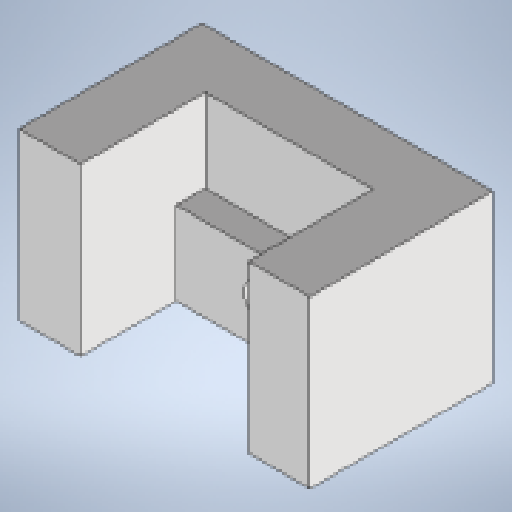
# Autodesk Inventor part: MotorMount
Saved by Autodesk Inventor 2026 (Build 300175050, 175E)
## iProperties
Created: 2025-12-25
Part Number: MotorMount
Material: Generic
Document SubType Name: Modeling
Designer: Nicholas M
Density: 1 g/cm^3
Appearance: Default
Author: Nicholas M
Autodesk Inventor part; units mm, degrees
ref_plane "YZ Plane" through (0, 0, 0) normal (1, 0, 0) x (0, 1, 0)
ref_plane "XZ Plane" through (0, 0, 0) normal (0, 1, 0) x (-1, 0, 0)
ref_plane "XY Plane" through (0, 0, 0) normal (0, 0, 1) x (1, 0, 0)
sketch "Sketch1" plane through (0, 16.25, -25.5) normal (1, 0, 0) x (0, 1, 0)
  line L0 (-35, 11.3959) -> (0, 11.3959)
  line L1 (0, 11.3959) -> (0, 41.3959)
  line L2 (0, 41.3959) -> (-35, 41.3959)
  line L3 (-35, 41.3959) -> (-35, 11.3959)
  line L4 (-17.5, 1.3959) -> (0, 1.3959)
  line L5 (-35, 41.3959) -> (0, 11.3959) construction
  line L6 (-35, 11.3959) -> (0, 41.3959) construction
  line L7 (-17.5, 53) -> (-17.5, 1.3959)
  circle A0 centre (-17.5, 16.3959) radius 2
  line L8 (-35, 26.3959) -> (0, 26.3959)
  line L9 (0, 26.3959) -> (0, 41.3959)
  line L10 (0, 41.3959) -> (-35, 41.3959)
  line L11 (-35, 41.3959) -> (-35, 26.3959)
  line L12 (-35, 11.3959) -> (-27.6, 11.3959)
  line L13 (-27.6, 11.3959) -> (-27.6, 41.3959)
  line L14 (-27.6, 41.3959) -> (-35, 41.3959)
  line L15 (-35, 41.3959) -> (-35, 11.3959)
  line L16 (0, 11.3959) -> (-7.4, 11.3959)
  line L17 (-7.4, 11.3959) -> (-7.4, 41.3959)
  line L18 (-7.4, 41.3959) -> (0, 41.3959)
  line L19 (0, 41.3959) -> (0, 11.3959)
  line L20 (0, 1.3959) -> (0, 49)
  line L21 (0, 31.3959) -> (0, 11.3959)
  line L22 (0, 11.3959) -> (0, 11.3959)
  line L23 (0, 11.3959) -> (0, 41.3959)
  line L24 (-35, 21.3959) -> (0, 21.3959)
  line L25 (-35, 18.8959) -> (-27.6, 18.8959)
  line L26 (-7.4, 18.8959) -> (0, 18.8959)
  line L27 (-35, 18.8959) -> (-27.6, 11.3959) construction
  line L28 (-35, 11.3959) -> (-27.6, 18.8959) construction
  circle A1 centre (-31.3, 15.1459) radius 1.625
  line L29 (-7.4, 11.3959) -> (0, 18.8959) construction
  line L30 (0, 11.3959) -> (-7.4, 18.8959) construction
  circle A2 centre (-3.7, 15.1459) radius 1.625
  line L31 (-35, 41.3959) -> (-27.6, 41.3959)
  line L32 (-27.6, 41.3959) -> (-27.6, 48.8959)
  line L33 (-27.6, 48.8959) -> (-35, 48.8959)
  line L34 (-35, 48.8959) -> (-35, 41.3959)
  line L35 (0, 41.3959) -> (-7.4, 41.3959)
  line L36 (-7.4, 41.3959) -> (-7.4, 48.8959)
  line L37 (-7.4, 48.8959) -> (0, 48.8959)
  line L38 (0, 48.8959) -> (0, 41.3959)
  line L39 (-35, 41.3959) -> (-27.6, 48.8959) construction
  line L40 (-35, 48.8959) -> (-27.6, 41.3959) construction
  line L41 (-7.4, 41.3959) -> (0, 48.8959) construction
  line L42 (-7.4, 48.8959) -> (0, 41.3959) construction
  circle A3 centre (-3.7, 45.1459) radius 1.625
  circle A4 centre (-31.3, 45.1459) radius 1.625
  circle A5 centre (-31.3, 30.1459) radius 2
  circle A6 centre (-3.7, 30.1459) radius 2
  line L43 (-27.6, 18.8959) -> (-35, 41.3959) construction
  line L44 (-35, 18.8959) -> (-27.6, 41.3959) construction
  point P0 (-17.5, 41.3959)
  point P1 (-17.5, 26.3959)
  point P2 (-1.25, 11.3959)
  point P3 (-27.6, 26.3959)
  point P4 (-7.4, 26.3959)
  point P5 (-7.4, 41.3959)
  point P6 (-7.4, 11.3959)
  point P7 (-27.6, 11.3959)
  point P8 (-17.5, 41.3959)
  point P9 (-17.5, 11.3959)
  point P10 (-1.25, 11.3959)
  point P11 (-7.4, 21.3959)
  point P12 (-27.6, 21.3959)
  point P13 (0, 21.3959)
  point P14 (0, 41.3959)
  point P15 (-3.7, 15.1459)
  dimension "d5" = 30
  dimension "d3" = 10
  dimension "d4" = 35
  dimension "d2" = 4
  dimension "d0" = 20.2
  dimension "d18" = 5
  dimension "d19" = 5
  dimension "d20" = 2.5
  dimension "d21" = 3.25
  dimension "d23" = 7.5
  dimension "d24" = 4
  dimension "d25" = 4
  constraints: 90 end point, 14 parallel, 13 point on line, 10 midpoint, 8 horizontal, 8 perpendicular, 7 centre point, 6 collinear, 3 equal radius, 2 vertical, 2 vertical alignment, 1 horizontal alignment
  measures "d5" distance of L0.end L1.end
  measures "d3" distance between parallel lines of L4 L0
  measures "d4" distance of L0.start L0.end
  measures "d2" diameter of A0
  measures "d0" distance between parallel lines of L17 L13
  measures "d18" distance from line of L0 A0.centre
  measures "d19" distance from line of A0.centre L24
  measures "d20" distance between parallel lines of L24 L26
  measures "d21" diameter of A1
  measures "d23" distance of L32.end L31.end
  measures "d24" diameter of A5
  measures "d25" diameter of A6
extrude "Extrusion1" add sketch "Sketch1" along normal blind 2 contours L3 L25 L13 L0 | L13 L24 L7 A0 L0 | L3 L24 L13 L25 | L7 A0 L24 L17 L0 | L3 L8 L13 L24 | L17 L26 L1 L0 | A0 L7 | L7 A0 | L13 L8 L7 L24 | L3 L2 L13 L8 | L17 L24 L1 L26 | L13 L2 L7 L8 | L7 L8 L17 L24 | L34 L33 L32 L2 | L17 L8 L1 L24 | L7 L2 L17 L8 | L17 L2 L1 L8 | L36 L37 L20 L2 | A5 | A6
extrude "Extrusion2" add sketch "Sketch1" along normal blind 1.5 from surface at 2 contours L3 L25 L13 L0 | L13 L24 L7 A0 L0 | L3 L24 L13 L25 | L7 A0 L24 L17 L0 | L3 L8 L13 L24 | L17 L26 L1 L0 | L13 L8 L7 L24 | L3 L2 L13 L8 | L17 L24 L1 L26 | L13 L2 L7 L8 | L7 L8 L17 L24 | L34 L33 L32 L2 | L17 L8 L1 L24 | L7 L2 L17 L8 | L17 L2 L1 L8 | L36 L37 L20 L2 | A5 | A6
extrude "Extrusion3" add sketch "Sketch1" along normal blind 3.5 from surface at 3.5 contours L13 L24 L7 A0 L0 | L7 A0 L24 L17 L0
extrude "Extrusion4" add sketch "Sketch1" along normal blind 15 from surface at 3.5 contours L3 L24 L13 L25 | L3 L8 L13 L24 | L3 L2 L13 L8 | L17 L24 L1 L26 | L17 L8 L1 L24 | L17 L2 L1 L8 | A5 | A6
fillet "Fillet1" radius 2 20 edges at (1.75, -18.75, -14.1041) (1.75, 16.25, -14.1041) (11, -18.75, -6.6041) (5.25, -11.35, -6.6041) (5.25, -11.35, -14.1041) (5.25, 8.85, -14.1041) (5.25, 8.85, -6.6041) (11, 16.25, -6.6041) (12.75, 8.85, -6.6041) (12.75, -11.35, -6.6041) (11, -11.35, 15.8959) (11, 8.85, 15.8959) (1.75, -18.75, 23.3959) (1.75, -11.35, 23.3959) (1.75, -11.35, 15.8959) (1.75, 8.85, 15.8959) (1.75, 8.85, 23.3959) (1.75, 16.25, 23.3959) (11, -18.75, 15.8959) (11, 16.25, 15.8959)
extrude "Extrusion5" cut sketch "Sketch1" against normal blind 5 from surface at 18.5 contours A5 | A6
body "Solid1"
